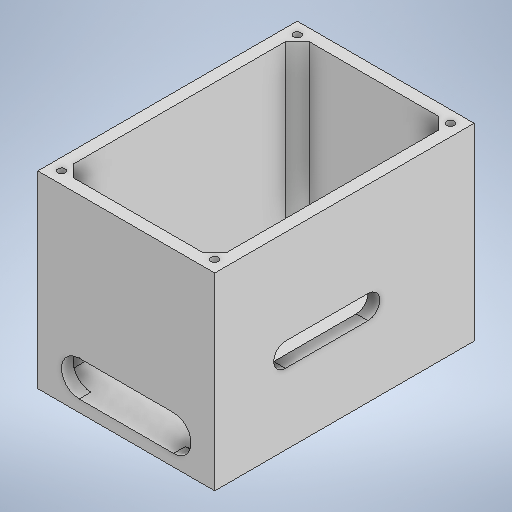
# Autodesk Inventor part: DAQ_Housing_V1
Saved by Autodesk Inventor 2025.2 (Build 292293000, 293)
## iProperties
Created: 2025-04-28
Part Number: DAQ_Housing_V1
Material: Generic
Document SubType Name: Modeling
Designer: limee
Density: 1 g/cm^3
Appearance: Default
Author: limee
Autodesk Inventor part; units mm, degrees
ref_plane "YZ Plane" through (0, 0, 0) normal (1, 0, 0) x (0, 1, 0)
ref_plane "XZ Plane" through (0, 0, 0) normal (0, 1, 0) x (-1, 0, 0)
ref_plane "XY Plane" through (0, 0, 0) normal (0, 0, 1) x (1, 0, 0)
sketch "Sketch1" plane through (0, 0, 0) normal (0, 1, 0) x (-1, 0, 0)
  line L0 (32.5, 50) -> (-32.5, 50)
  line L1 (-32.5, 50) -> (-32.5, -50)
  line L2 (-32.5, -50) -> (32.5, -50)
  line L3 (32.5, -50) -> (32.5, 50)
  line L4 (32.5, 50) -> (-32.5, -50) construction
  line L5 (-32.5, 50) -> (32.5, -50) construction
  line L6 (37.5, -55) -> (-37.5, -55)
  line L7 (-37.5, -55) -> (-37.5, 55)
  line L8 (-37.5, 55) -> (37.5, 55)
  line L9 (37.5, 55) -> (37.5, -55)
  line L10 (-32.5, 45) -> (-27.5, 50)
  line L11 (-32.5, 45) -> (-25.4289, 45) construction
  line L12 (0, 55) -> (0, -55) construction
  line L13 (-37.5, 0) -> (37.5, 0) construction
  line L14 (32.5, 45) -> (27.5, 50)
  line L15 (-32.5, -45) -> (-27.5, -50)
  line L16 (32.5, -45) -> (27.5, -50)
  point P0 (0, 0)
  dimension "d0" = 100
  dimension "d1" = 65
  dimension "d2" = 5
  dimension "d29" = 45
  dimension "d30" = 5
  constraints: 34 end point, 6 midpoint, 6 symmetric about line, 4 parallel, 2 horizontal, 2 perpendicular, 2 point on line, 1 equal length, 3 other
  measures "d0" distance of L0.end L1.end
  measures "d1" distance of L0.start L0.end
  measures "d2" distance between parallel lines of L6 L2
  measures "d29" angle of L11 L10
  measures "d30" distance from line of L10.start L0
extrude "Extrusion1" add sketch "Sketch1" along normal blind 80 contours L3 L14 L0 | L10 L1 L0 | L3 L2 L16 | L15 L2 L1 | L6 L7 L8 L9
extrude "Extrusion2" add sketch "Sketch1" along normal blind 5 contours L3 L14 L0 | L14 L3 L16 L2 L15 L1 L10 L0 | L10 L1 L0 | L3 L2 L16 | L15 L2 L1
sketch "Sketch3" plane through (37.5, 0, 55) normal (1, 0, 0) x (0, 0, -1)
  line L0 (30, 40) -> (65, 40) construction
  line L1 (65, 40) -> (65, 30) construction
  line L2 (65, 30) -> (30, 30) construction
  line L3 (30, 30) -> (30, 40) construction
  line L4 (30, 40) -> (65, 30) construction
  line L5 (65, 40) -> (30, 30) construction
  line L6 (0, 0) -> (110, 0) projected
  line L7 (0, 0) -> (0, 80) projected
  line L8 (30, 35) -> (65, 35) construction
  line L9 (30, 30) -> (65, 30)
  line L10 (65, 40) -> (30, 40)
  arc A0 (30, 40) -> (30, 30) centre (30, 35) ccw
  arc A1 (65, 30) -> (65, 40) centre (65, 35) ccw
  point P0 (55, 0)
  point P1 (47.5, 35)
  point P2 (47.5, 40)
  dimension "d12" = 30
  dimension "d13" = 10
  dimension "d14" = 30
  dimension "d15" = 35
  constraints: 20 end point, 6 midpoint, 4 point on circle, 4 tangent, 3 parallel, 2 centre point, 1 horizontal, 1 perpendicular
  measures "d12" distance between parallel lines of L2 L6
  measures "d13" distance between parallel lines of L2 L0
  measures "d14" distance between parallel lines of L7 L3
  measures "d15" distance between parallel lines of L3 L1
extrude "Extrusion4" cut sketch "Sketch3" against normal up to next
sketch "Sketch4" plane through (0, 80, 0) normal (0, 1, 0) x (1, 0, 0)
  line L0 (-37.5, -55) -> (37.5, -55) projected
  line L1 (37.5, -55) -> (37.5, 55) projected
  line L2 (37.5, 55) -> (-37.5, 55) projected
  line L3 (-37.5, 55) -> (-37.5, -55) projected
  point P0 (0, 0)
  point P1 (-32.5, -50)
  point P2 (-32.5, 50)
  point P3 (32.5, 50)
  point P4 (32.5, -50)
  dimension "d25" = 5
  dimension "d26" = 5
  dimension "d27" = 5
  dimension "d28" = 5
  constraints: 2 horizontal alignment, 2 vertical alignment
  measures "d25" distance from line of point (32.5, -50) L0
  measures "d26" distance from line of L1 point (32.5, -50)
  measures "d27" distance from line of L2 point (32.5, 50)
  measures "d28" distance from line of L3 point (-32.5, -50)
hole "Hole1" at (-32.5, 80, 50) at (-32.5, 80, -50) at (32.5, 80, -50) at (32.5, 80, 50) direction (0, -1, 0) diameter 3.2 depth 6
sketch "Sketch5" plane through (-37.5, 0, 55) normal (0, 0, 1) x (1, 0, 0)
  line L0 (65, 5) -> (10, 5) projected
  line L1 (17.5, 12.5) -> (57.5, 12.5) construction
  line L2 (17.5, 20) -> (57.5, 20)
  line L3 (57.5, 5) -> (17.5, 5)
  arc A0 (17.5, 20) -> (17.5, 5) centre (17.5, 12.5) ccw
  arc A1 (57.5, 5) -> (57.5, 20) centre (57.5, 12.5) ccw
  line L4 (10, 5) -> (10, 80) projected
  line L5 (65, 5) -> (65, 80) projected
  point P0 (37.5, 0)
  point P1 (37.5, 12.5)
  point P2 (37.5, 5)
  point P3 (10, 12.5)
  point P4 (65, 12.5)
  dimension "d31" = 15
  constraints: 8 end point, 6 point on circle, 4 tangent, 3 midpoint, 2 centre point, 2 parallel, 2 point on line
  measures "d31" distance between parallel lines of L2 L0
extrude "Extrusion5" cut sketch "Sketch5" against normal up to next contours L0 A0 L2 A1
body "Solid1"
